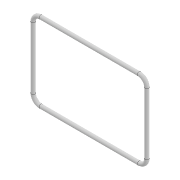
# Autodesk Inventor part: O-RING DASH 034
Saved by Autodesk Inventor 2020 (Build 240168000, 168)
## iProperties
Created: 2020-04-15
Part Number: O-RING DASH 034
Material: Generic
Document SubType Name: Modeling
Designer: John K
Density: 1 g/cm^3
Appearance: Default
Description: McM 9452K122
Author: John K
Autodesk Inventor part; units mm, degrees
ref_plane "YZ Plane" through (0, 0, 0) normal (1, 0, 0) x (0, 1, 0)
ref_plane "XZ Plane" through (0, 0, 0) normal (0, 1, 0) x (-1, 0, 0)
ref_plane "XY Plane" through (0, 0, 0) normal (0, 0, 1) x (1, 0, 0)
sketch "Sketch1" plane through (0, 0, 0) normal (0, 0, 1) x (1, 0, 0)
  line L0 (-26.875, -18.2565) -> (26.875, -18.2565) construction
  line L1 (26.875, -18.2565) -> (26.875, 18.2565) construction
  line L2 (26.875, 18.2565) -> (-26.875, 18.2565) construction
  line L3 (-26.875, 18.2565) -> (-26.875, -18.2565) construction
  line L4 (-27.764, 19.1455) -> (27.764, 19.1455)
  line L5 (27.764, 19.1455) -> (27.764, -19.1455)
  line L6 (27.764, -19.1455) -> (-27.764, -19.1455)
  line L7 (-27.764, -19.1455) -> (-27.764, 19.1455)
  line L8 (-25.986, 17.3675) -> (25.986, 17.3675)
  line L9 (25.986, 17.3675) -> (25.986, -17.3675)
  line L10 (25.986, -17.3675) -> (-25.986, -17.3675)
  line L11 (-25.986, -17.3675) -> (-25.986, 17.3675)
  point P0 (0, 0)
  point P1 (0, 18.2565)
  point P2 (-26.875, 0)
  dimension "d0" = 53.75
  dimension "d1" = 36.513
  dimension "d2" = 0.889
  dimension "d3" = 0.889
  constraints: 24 end point, 6 parallel, 3 perpendicular, 2 midpoint, 1 horizontal, 1 horizontal alignment, 1 vertical alignment, 6 other
  measures "d0" distance of L1.end L2.end
  measures "d1" distance of L0.end L1.end
  measures "d2" distance between parallel lines of L2 L4
  measures "d3" distance between parallel lines of L2 L8
extrude "Extrusion1" add sketch "Sketch1" along normal mid plane 1.778
fillet "Fillet1" radius 4.535 4 edges at (27.764, 19.1455, 0) (27.764, -19.1455, 0) (-27.764, -19.1455, 0) (-27.764, 19.1455, 0)
sketch "Sketch2" plane through (0, 0, 0.889) normal (0, 0, 1) x (1, 0, 0)
  arc A0 (-23.229, 19.1455) -> (-27.764, 14.6105) centre (-23.229, 14.6105) ccw projected
  line L0 (-27.764, 14.6105) -> (-27.764, -14.6105) projected
  arc A1 (-27.764, -14.6105) -> (-23.229, -19.1455) centre (-23.229, -14.6105) ccw projected
  line L1 (-23.229, -19.1455) -> (23.229, -19.1455) projected
  arc A2 (23.229, -19.1455) -> (27.764, -14.6105) centre (23.229, -14.6105) ccw projected
  line L2 (27.764, -14.6105) -> (27.764, 14.6105) projected
  arc A3 (27.764, 14.6105) -> (23.229, 19.1455) centre (23.229, 14.6105) ccw projected
  line L3 (23.229, 19.1455) -> (-23.229, 19.1455) projected
  line L4 (-25.986, -17.3675) -> (-25.986, 17.3675) projected
  line L5 (-25.986, 17.3675) -> (25.986, 17.3675) projected
  line L6 (25.986, 17.3675) -> (25.986, -17.3675) projected
  line L7 (25.986, -17.3675) -> (-25.986, -17.3675) projected
  line L8 (-25.986, 17.3675) -> (25.986, 17.3675) projected
  arc A4 (-23.229, 17.3675) -> (-25.986, 14.6105) centre (-23.229, 14.6105) ccw
  line L9 (25.986, 17.3675) -> (25.986, -17.3675) projected
  arc A5 (25.986, 14.6105) -> (23.229, 17.3675) centre (23.229, 14.6105) ccw
  line L10 (-25.986, -17.3675) -> (-25.986, 17.3675) projected
  line L11 (25.986, -17.3675) -> (-25.986, -17.3675) projected
  arc A6 (-25.986, -14.6105) -> (-23.229, -17.3675) centre (-23.229, -14.6105) ccw
  arc A7 (23.229, -17.3675) -> (25.986, -14.6105) centre (23.229, -14.6105) ccw
  point P0 (0, 0)
  point P1 (23.229, 17.3675)
  point P2 (-23.229, 17.3675)
  constraints: 8 point on circle, 8 point on line, 8 tangent, 4 centre point, 4 coincident
extrude "Extrusion2" add sketch "Sketch2" against normal blind 1.778 contours L4 A6 L7 | L4 L5 A4 | A7 L6 L7 | L5 L6 A5
fillet "Fillet2" radius 0.889 32 edges at (25.1785, 16.56, 0.889) (25.986, 0, 0.889) (25.1785, -16.56, 0.889) (0, -17.3675, 0.889) (-25.1785, -16.56, 0.889) (-25.986, 0, 0.889) (-25.1785, 16.56, 0.889) (0, 17.3675, 0.889) (-26.4357, -17.8172, 0.889) (0, -19.1455, 0.889) (26.4357, -17.8172, 0.889) (27.764, 0, 0.889) (26.4357, 17.8172, 0.889) (0, 19.1455, 0.889) (-26.4357, 17.8172, 0.889) (-27.764, 0, 0.889) (-26.4357, 17.8172, -0.889) (0, 19.1455, -0.889) (26.4357, 17.8172, -0.889) (27.764, 0, -0.889) (26.4357, -17.8172, -0.889) (0, -19.1455, -0.889) (-26.4357, -17.8172, -0.889) (-27.764, 0, -0.889) (-25.1785, -16.56, -0.889) (0, -17.3675, -0.889) (25.1785, -16.56, -0.889) (25.986, 0, -0.889) (25.1785, 16.56, -0.889) (0, 17.3675, -0.889) (-25.1785, 16.56, -0.889) (-25.986, 0, -0.889)
equation "\"d3\" = d2"
equation "\"d4\" = 2 * d2"
equation "\"d7\" = 2 * d2"
equation "\"d9\" = d2"
body "Solid1"
